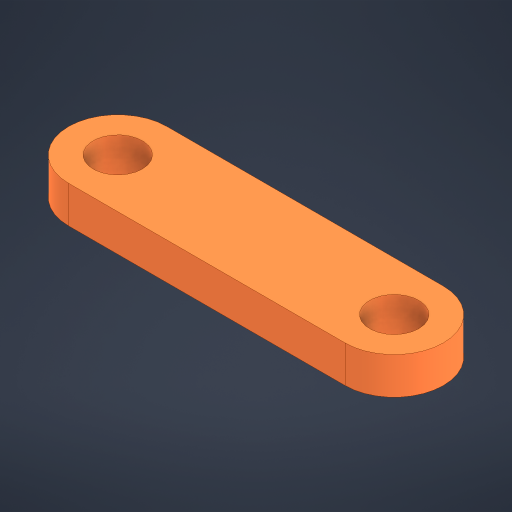
# Autodesk Inventor part: side
Saved by Autodesk Inventor 2024 (Build 280153000, 153)
## iProperties
Created: 2023-05-10
Part Number: side
Material: Типовые
Document SubType Name: Modeling
Designer: user
Density: 1 g/cm^3
Appearance: По умолчанию
Author: user
Autodesk Inventor part; units mm, degrees
ref_plane "YZ Plane" through (0, 0, 0) normal (1, 0, 0) x (0, 1, 0)
ref_plane "XZ Plane" through (0, 0, 0) normal (0, 1, 0) x (-1, 0, 0)
ref_plane "XY Plane" through (0, 0, 0) normal (0, 0, 1) x (1, 0, 0)
sketch "Эскиз1" plane through (0, 0, 0) normal (0, 0, 1) x (1, 0, 0)
  circle A0 centre (0, 0) radius 2
  arc A1 (0, 4) -> (0, -4) centre (0, 0) ccw
  line L0 (0, 4) -> (22.5, 4)
  line L1 (0, -4) -> (22.5, -4)
  arc A2 (22.5, -4) -> (22.5, 4) centre (22.5, 0) ccw
  circle A3 centre (22.5, 0) radius 2
  point P0 (26.5, 0)
  point P1 (-4, 0)
  dimension "d0" = 8
  dimension "d1" = 4
  dimension "d2" = 22.5
  constraints: 6 point on circle, 4 centre point, 4 end point, 4 tangent, 3 coincident, 2 horizontal, 2 horizontal alignment, 1 equal radius
  measures "d0" distance of L1.start L0.start
  measures "d1" diameter of A3
  measures "d2" distance of A2.centre point (0, 0)
extrude "Выдавливание1" add sketch "Эскиз1" along normal blind 3
